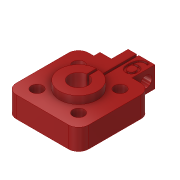
# Autodesk Inventor part: clamping hub 6mm round nut wells shortened clamp
Saved by Autodesk Inventor 2020 (Build 240168000, 168)
## iProperties
Created: 2019-10-18
Part Number: clamping hub 6mm round nut wells shortened clamp
Material: Generic
Document SubType Name: Modeling
Designer: ball
Density: 1 g/cm^3
Appearance: Default
Author: ball
Autodesk Inventor part; units mm, degrees
ref_plane "YZ Plane" through (0, 0, 0) normal (1, 0, 0) x (0, 1, 0)
ref_plane "XZ Plane" through (0, 0, 0) normal (0, 1, 0) x (-1, 0, 0)
ref_plane "XY Plane" through (0, 0, 0) normal (0, 0, 1) x (1, 0, 0)
sketch "Sketch1" plane through (0, 0, 0) normal (0, 1, 0) x (-1, 0, 0)
  line L0 (-12.065, 12.065) -> (12.065, 12.065)
  line L1 (12.065, 12.065) -> (12.065, -12.065)
  line L2 (-12.065, -12.065) -> (-12.065, 12.065)
  circle A0 centre (6.9148, -6.9148) radius 1.9304
  circle A1 centre (6.9148, 6.9148) radius 1.9304
  circle A2 centre (-6.9148, 6.9148) radius 1.9304
  circle A3 centre (-6.9148, -6.9148) radius 1.9304
  line L3 (-5.715, -12.065) -> (-5.715, -19.685)
  line L4 (-5.715, -19.685) -> (6.985, -19.685)
  line L5 (6.985, -19.685) -> (6.985, -12.065)
  line L6 (12.065, -12.065) -> (6.985, -12.065)
  line L7 (-5.715, -12.065) -> (-12.065, -12.065)
  point P0 (0, 0)
  dimension "d0" = 24.13
  dimension "d2" = 12.065
  dimension "d3" = 12.065
  dimension "d4" = 3.8608
  dimension "d5" = 6.9148
  dimension "d6" = 6.9148
  dimension "d7" = 3.8608
  dimension "d8" = 6.9148
  dimension "d9" = 6.9148
  dimension "d10" = 3.8608
  dimension "d11" = 6.9148
  dimension "d12" = 6.9148
  dimension "d13" = 3.8608
  dimension "d14" = 12.7
  dimension "d16" = 6.985
  dimension "d41" = 6.9148
  dimension "d42" = 6.9148
  dimension "d43" = 24.13
  dimension "d44" = 24.13
  dimension "d50" = 7.62
  dimension "d51" = 7.62
  constraints: 16 end point, 4 centre point, 4 parallel, 1 horizontal, 1 perpendicular
  measures "d0" distance of L1.end L2.start
  measures "d2" distance from line of L0 point (0, 0)
  measures "d3" distance from line of L1 point (0, 0)
  measures "d4" diameter of A0
  measures "d5" horizontal distance of A0.centre point (0, 0)
  measures "d6" horizontal distance of A0.centre point (0, 0)
  measures "d7" diameter of A1
  measures "d8" horizontal distance of point (0, 0) A1.centre
  measures "d9" horizontal distance of point (0, 0) A1.centre
  measures "d10" diameter of A2
  measures "d11" horizontal distance of point (0, 0) A2.centre
  measures "d12" horizontal distance of A2.centre point (0, 0)
  measures "d13" diameter of A3
  measures "d14" distance of L4.end L3.end
  measures "d16" distance from line of L5 point (0, 0)
  measures "d41" horizontal distance of A3.centre point (0, 0)
  measures "d42" horizontal distance of A3.centre point (0, 0)
  measures "d43" distance between parallel lines of L7 L0
  measures "d44" distance between parallel lines of L6 L0
  measures "d50" distance between parallel lines of L7 L4
  measures "d51" distance between parallel lines of L6 L4
extrude "Shape" add sketch "Sketch1" along normal blind 6.985
sketch "Sketch2" plane through (-6.985, 0, -19.685) normal (-1, 0, 0) x (0, 0, 1)
  circle A0 centre (2.921, 3.4925) radius 4.6609 construction
  line L0 (7.62, 0) -> (0, 0) projected
  line L1 (0, 0) -> (0, 6.985) projected
  line L2 (7.5819, 3.4925) -> (5.2514, -0.544)
  line L3 (5.2514, -0.544) -> (0.5905, -0.544)
  line L4 (0.5905, -0.544) -> (-1.7399, 3.4925)
  line L5 (-1.7399, 3.4925) -> (0.5905, 7.529)
  line L6 (0.5905, 7.529) -> (5.2514, 7.529)
  line L7 (5.2514, 7.529) -> (7.5819, 3.4925)
  line L8 (7.62, 0) -> (7.62, 6.985) projected
  point P0 (19.685, 0)
  dimension "d19" = 9.3218
  dimension "d20" = 3.4925
  dimension "d52" = 4.699
  constraints: 12 end point, 1 coincident, 1 horizontal alignment, 15 other
  measures "d20" distance from line of L0 point (2.921, 3.493)
  measures "d52" distance from line of L8 point (2.921, 3.493)
extrude "NutWellSide" cut sketch "Sketch2" against normal blind 3.81 contours L2 L3 L4 L0 | L0 L4 L1 L5 L6 L7 L2 | L4 L5 L1
sketch "Sketch3" plane through (5.715, 0, -12.065) normal (1, 0, 0) x (0, 0, -1)
  circle A0 centre (4.699, 3.4925) radius 1.9304
  line L0 (7.62, 0) -> (7.62, 6.985) projected
  line L1 (0, 6.985) -> (7.62, 6.985) projected
  line L2 (0, 0) -> (0, 6.985) projected
  point P0 (-12.065, 0)
  dimension "d24" = 3.8608
  dimension "d26" = 3.4925
  dimension "d53" = 4.699
  constraints: 1 centre point
  measures "d24" diameter of A0
  measures "d26" distance from line of L1 A0.centre
  measures "d53" distance from line of L2 A0.centre
extrude "HoleClamping" cut sketch "Sketch3" against normal through all
sketch "Sketch4" plane through (0, 6.985, 0) normal (0, 1, 0) x (1, 0, 0)
  circle A0 centre (0, 0) radius 6.35
  dimension "d29" = 12.7
  constraints: 1 centre point, 1 coincident
  measures "d29" diameter of A0
extrude "Boss" add sketch "Sketch4" along normal blind 2.54
sketch "Sketch5" plane through (0, 9.525, 0) normal (0, 1, 0) x (1, 0, 0)
  circle A0 centre (0, 0) radius 3.15
  dimension "d60" = 6.3
  constraints: 1 centre point, 1 coincident
  measures "d60" diameter of A0
fillet "Fillet1" radius 3.3782 4 edges at (12.065, 3.4925, 12.065) (12.065, 3.4925, -12.065) (-12.065, 3.4925, 12.065) (-12.065, 3.4925, -12.065)
extrude "HoleD" cut sketch "Sketch5" against normal through all
sketch "Sketch6" plane through (0, 9.525, 0) normal (0, 1, 0) x (1, 0, 0)
  line L0 (-6.985, 19.685) -> (5.715, 19.685) projected
  line L1 (5.715, 19.685) -> (-6.985, 19.685) projected
  line L2 (-0.381, 0) -> (0.381, 0)
  line L3 (0.381, 0) -> (0.381, 19.685)
  line L4 (0.381, 19.685) -> (-0.381, 19.685)
  line L5 (-0.381, 19.685) -> (-0.381, 0)
  line L6 (0, 26.035) -> (0, -18.415) projected
  point P0 (0, 0)
  point P1 (-3.175, 19.177)
  point P2 (-0.127, 0)
  dimension "d56" = 0.762
  dimension "d57" = 0.381
  constraints: 8 end point, 2 parallel, 2 point on line, 1 horizontal, 1 perpendicular, 2 other
  measures "d56" distance of L4.end L3.end
  measures "d57" distance of the line from the sketch origin of L3
extrude "ClampingSlot" cut sketch "Sketch6" against normal through all
sketch "Sketch7" plane through (0, 0, 0) normal (0, -1, 0) x (1, 0, 0)
  circle A0 centre (-6.9148, 6.9148) radius 1.9304 construction
  circle A1 centre (-6.9148, 6.9148) radius 4.6609 construction
  line L0 (-6.9148, 2.2539) -> (-10.9513, 4.5843)
  line L1 (-10.9513, 4.5843) -> (-10.9513, 9.2452)
  line L2 (-10.9513, 9.2452) -> (-6.9148, 11.5757)
  line L3 (-6.9148, 11.5757) -> (-2.8783, 9.2452)
  line L4 (-2.8783, 9.2452) -> (-2.8783, 4.5843)
  line L5 (-2.8783, 4.5843) -> (-6.9148, 2.2539)
  circle A2 centre (-6.9148, -6.9148) radius 1.9304 construction
  circle A3 centre (-6.9148, -6.9148) radius 4.6609 construction
  circle A4 centre (6.9148, -6.9148) radius 1.9304 construction
  circle A5 centre (6.9148, -6.9148) radius 4.6609 construction
  circle A6 centre (6.9148, 6.9148) radius 1.9304 construction
  circle A7 centre (6.9148, 6.9148) radius 4.6609 construction
  line L6 (6.9148, 2.2539) -> (2.8783, 4.5843)
  line L7 (2.8783, 4.5843) -> (2.8783, 9.2452)
  line L8 (2.8783, 9.2452) -> (6.9148, 11.5757)
  line L9 (6.9148, 11.5757) -> (10.9513, 9.2452)
  line L10 (10.9513, 9.2452) -> (10.9513, 4.5843)
  line L11 (10.9513, 4.5843) -> (6.9148, 2.2539)
  line L12 (6.9148, -2.2539) -> (10.9513, -4.5843)
  line L13 (10.9513, -4.5843) -> (10.9513, -9.2452)
  line L14 (10.9513, -9.2452) -> (6.9148, -11.5757)
  line L15 (6.9148, -11.5757) -> (2.8783, -9.2452)
  line L16 (2.8783, -9.2452) -> (2.8783, -4.5843)
  line L17 (2.8783, -4.5843) -> (6.9148, -2.2539)
  line L18 (-6.9148, -2.2539) -> (-2.8783, -4.5843)
  line L19 (-2.8783, -4.5843) -> (-2.8783, -9.2452)
  line L20 (-2.8783, -9.2452) -> (-6.9148, -11.5757)
  line L21 (-6.9148, -11.5757) -> (-10.9513, -9.2452)
  line L22 (-10.9513, -9.2452) -> (-10.9513, -4.5843)
  line L23 (-10.9513, -4.5843) -> (-6.9148, -2.2539)
  point P0 (0, 0)
  dimension "d40" = 9.3218
  dimension "d45" = 9.3218
  dimension "d46" = 9.3218
  dimension "d47" = 9.3218
  constraints: 48 end point, 8 coincident, 4 vertical alignment, 60 other
extrude "NutWellAttachment" cut sketch "Sketch7" against normal blind 3.048
sketch "Sketch8" plane through (-3.175, 0.4789, -19.685) normal (0, 0, -1) x (-1, 0, 0)
  line L0 (-11.8618, -0.4789) -> (5.5118, -0.4789) projected
  line L1 (3.81, -0.4789) -> (3.81, 6.5061) projected
  line L2 (0, -0.4789) -> (3.81, -0.4789)
  line L3 (3.81, -0.4789) -> (3.81, 6.5061)
  line L4 (3.81, 6.5061) -> (0, 6.5061)
  line L5 (0, 6.5061) -> (0, -0.4789)
  point P0 (-3.175, -0.4789)
  constraints: 8 end point, 2 parallel, 1 horizontal, 1 perpendicular, 1 point on line
extrude "Extrusion8" cut sketch "Sketch8" against normal blind 0.635
sketch "Sketch9" plane through (0, 6.985, 0) normal (0, 1, 0) x (1, 0, 0)
  line L0 (0.6918, 19.0045) -> (5.4568, 19.0045) construction
  line L1 (5.4568, 19.0045) -> (5.4568, 12.6545) construction
  line L2 (5.4568, 12.6545) -> (0.6918, 12.6545) construction
  line L3 (0.6918, 12.6545) -> (0.6918, 19.0045) construction
  spline S0 degree 2 poles (5.1687, 14.7205) (5.1687, 14.2317) (4.8445, 13.4032) (4.5718, 13.1253) knots 0 0 0 1 2 2 2
  spline S1 degree 2 poles (4.5718, 13.1253) (4.2887, 12.832) (3.5786, 12.5284) (3.1515, 12.5284) knots 0 0 0 1 2 2 2
  spline S2 degree 2 poles (3.1515, 12.5284) (2.7244, 12.5284) (2.0194, 12.8166) (1.7518, 13.1047) knots 0 0 0 1 2 2 2
  spline S3 degree 2 poles (1.7518, 13.1047) (1.4225, 13.4495) (1.052, 14.6073) (1.052, 15.4512) knots 0 0 0 1 2 2 2
  spline S4 degree 2 poles (1.052, 15.4512) (1.052, 16.2797) (1.3916, 17.6125) (1.7467, 18.1065) knots 0 0 0 1 2 2 2
  spline S5 degree 2 poles (1.7467, 18.1065) (2.0915, 18.5902) (3.1824, 19.1305) (3.8977, 19.1305) knots 0 0 0 1 2 2 2
  spline S6 degree 2 poles (3.8977, 19.1305) (4.1086, 19.1305) (4.4791, 19.0894) (4.6181, 19.0431) knots 0 0 0 1 2 2 2
  line L4 (4.6181, 19.0431) -> (4.6181, 18.2249)
  line L5 (4.6181, 18.2249) -> (4.5821, 18.2249)
  spline S7 degree 2 poles (4.5821, 18.2249) (4.4637, 18.2866) (4.0314, 18.3947) (3.7844, 18.3947) knots 0 0 0 1 2 2 2
  spline S8 degree 2 poles (3.7844, 18.3947) (2.992, 18.3947) (2.0194, 17.3243) (1.9268, 16.2746) knots 0 0 0 1 2 2 2
  spline S9 degree 2 poles (1.9268, 16.2746) (2.2304, 16.4856) (2.8685, 16.7171) (3.2493, 16.7171) knots 0 0 0 1 2 2 2
  spline S10 degree 2 poles (3.2493, 16.7171) (3.6198, 16.7171) (4.1755, 16.5679) (4.4791, 16.3415) knots 0 0 0 1 2 2 2
  spline S11 degree 2 poles (4.4791, 16.3415) (4.8291, 16.079) (5.1687, 15.266) (5.1687, 14.7205) knots 0 0 0 1 2 2 2
  spline S12 degree 2 poles (4.3042, 14.6845) (4.3042, 15.0756) (4.0983, 15.6056) (3.8719, 15.7909) knots 0 0 0 1 2 2 2
  spline S13 degree 2 poles (3.8719, 15.7909) (3.7021, 15.9247) (3.2801, 16.0121) (3.0589, 16.0121) knots 0 0 0 1 2 2 2
  spline S14 degree 2 poles (3.0589, 16.0121) (2.7604, 16.0121) (2.1995, 15.832) (1.9268, 15.6622) knots 0 0 0 1 2 2 2
  spline S15 degree 2 poles (1.9268, 15.6622) (1.9216, 15.5696) (1.9113, 15.3946) (1.9113, 15.2608) knots 0 0 0 1 2 2 2
  spline S16 degree 2 poles (1.9113, 15.2608) (1.9113, 14.6022) (2.1686, 13.7943) (2.3642, 13.5833) knots 0 0 0 1 2 2 2
  spline S17 degree 2 poles (2.3642, 13.5833) (2.5443, 13.3826) (2.9354, 13.2231) (3.1566, 13.2231) knots 0 0 0 1 2 2 2
  spline S18 degree 2 poles (3.1566, 13.2231) (3.6712, 13.2231) (4.3042, 13.9538) (4.3042, 14.6845) knots 0 0 0 1 2 2 2
  point P0 (0, 0)
  constraints: 2 other
emboss "Emboss1" sketch "Sketch9" operation cut depth 0.635 direction (0, -1, 0)
equation "\"d2\" = 0.5 * d0"
equation "\"d3\" = 0.5 * d0"
equation "\"d7\" = d4"
equation "\"d8\" = d9"
equation "\"d9\" = d5"
equation "\"d10\" = d4"
equation "\"d11\" = d9"
equation "\"d12\" = d9"
equation "\"d13\" = d4"
equation "\"d41\" = d9"
equation "\"d42\" = d5"
equation "\"d43\" = d0"
equation "\"d44\" = d0"
equation "\"d57\" = 0.5 * d56"
equation "\"d6\" = d9"
body "Solid1"
